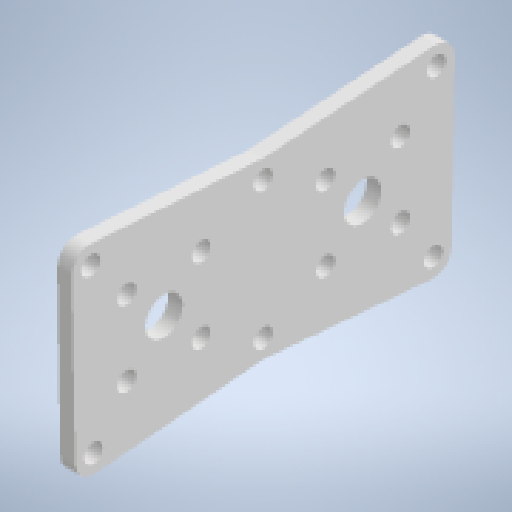
# Autodesk Inventor part: motorMountPlate2.0
Saved by Autodesk Inventor 2023 (Build 270158000, 158)
## iProperties
Created: 2022-09-08
Part Number: motorMountPlate2.0
Material: Generic
Document SubType Name: Modeling
Designer: deli
Density: 1 g/cm^3
Appearance: Default
Author: deli
Autodesk Inventor part; units mm, degrees
ref_plane "YZ Plane" through (0, 0, 0) normal (1, 0, 0) x (0, 1, 0)
ref_plane "XZ Plane" through (0, 0, 0) normal (0, 1, 0) x (-1, 0, 0)
ref_plane "XY Plane" through (0, 0, 0) normal (0, 0, 1) x (1, 0, 0)
sketch "Sketch1" plane through (0, 0, 0) normal (1, 0, 0) x (0, 1, 0)
  circle A0 centre (47.4062, -13.6361) radius 2 projected
  circle A1 centre (14.2614, -11.9601) radius 2 projected
  circle A2 centre (15.5288, -50.354) radius 2 projected
  circle A3 centre (44.494, -50.354) radius 2 projected
  circle A4 centre (47.4062, -87.072) radius 2 projected
  circle A5 centre (14.2614, -88.7479) radius 2 projected
  circle A6 centre (30.0114, -29.0628) radius 7 construction
  circle A7 centre (30.0114, -71.6453) radius 7 construction
  circle A8 centre (30.0114, -29.0628) radius 4
  circle A9 centre (30.0114, -71.6453) radius 4
  circle A10 centre (30.0114, -29.0628) radius 9.3137 construction
  circle A11 centre (30.0114, -71.6453) radius 9.3137 construction
  arc A12 (51.3935, -13.9551) -> (47.6082, -9.6412) centre (47.4062, -13.6361) ccw
  circle A13 centre (44.494, -50.354) radius 4 construction
  circle A14 centre (15.5288, -50.354) radius 4 construction
  arc A15 (14.4634, -7.9653) -> (10.2636, -12.0926) centre (14.2614, -11.9601) ccw
  arc A16 (10.2636, -88.6155) -> (14.4634, -92.7428) centre (14.2614, -88.7479) ccw
  arc A17 (47.6082, -91.0669) -> (51.3935, -86.7529) centre (47.4062, -87.072) ccw
  arc A18 (48.5067, -50.035) -> (48.5067, -50.6731) centre (52.494, -50.354) ccw
  arc A19 (11.5266, -50.4865) -> (11.5266, -50.2216) centre (7.5288, -50.354) ccw
  circle A20 centre (38.0114, -21.0628) radius 2
  circle A21 centre (38.0114, -37.0628) radius 2
  circle A22 centre (22.0114, -21.0628) radius 2
  circle A23 centre (22.0114, -37.0628) radius 2
  circle A24 centre (22.0114, -63.6453) radius 2
  circle A25 centre (22.0114, -79.6453) radius 2
  circle A26 centre (38.0114, -79.6453) radius 2
  circle A27 centre (38.0114, -63.6453) radius 2
  line L0 (38.0114, -21.0628) -> (38.0114, -37.0628) construction
  line L1 (38.0114, -37.0628) -> (22.0114, -37.0628) construction
  line L2 (22.0114, -37.0628) -> (22.0114, -21.0628) construction
  line L3 (22.0114, -21.0628) -> (38.0114, -21.0628) construction
  line L4 (38.0114, -63.6453) -> (38.0114, -79.6453) construction
  line L5 (38.0114, -79.6453) -> (22.0114, -79.6453) construction
  line L6 (22.0114, -79.6453) -> (22.0114, -63.6453) construction
  line L7 (38.0114, -63.6453) -> (22.0114, -63.6453) construction
  line L8 (51.3935, -13.9551) -> (48.5067, -50.035)
  line L9 (48.5067, -50.6731) -> (51.3935, -86.7529)
  line L10 (47.6082, -91.0669) -> (14.4634, -92.7428)
  line L11 (10.2636, -88.6155) -> (11.5266, -50.4865)
  line L12 (11.5266, -50.2216) -> (10.2636, -12.0926)
  line L13 (14.4634, -7.9653) -> (47.6082, -9.6412)
  point P0 (0, 0)
  dimension "d0" = 8
  dimension "d1" = 8
  dimension "d2" = 8
  dimension "d3" = 8
  dimension "d4" = 8
  dimension "d5" = 8
  dimension "d6" = 8
  dimension "d7" = 0
  dimension "d8" = 8
  dimension "d9" = 0
  dimension "d10" = 4
  dimension "d11" = 4
  dimension "d12" = 4
  dimension "d13" = 4
  dimension "d14" = 4
  dimension "d15" = 4
  dimension "d16" = 4
  dimension "d17" = 4
  dimension "d18" = 8
  dimension "d19" = 8
  dimension "d20" = 16
  dimension "d21" = 16
  dimension "d22" = 16
  dimension "d23" = 16
  constraints: 28 end point, 22 tangent, 20 centre point, 12 point on circle, 10 coincident, 3 perpendicular, 2 vertical, 1 collinear
  measures "d0" diameter of A12
  measures "d1" diameter of A18
  measures "d2" diameter of A15
  measures "d3" diameter of A14
  measures "d4" diameter of A19
  measures "d5" diameter of A16
  measures "d6" diameter of A17
  measures "d7" vertical distance of A18.centre A3.centre
  measures "d8" diameter of A13
  measures "d9" vertical distance of A14.centre A19.centre
  measures "d10" diameter of A22
  measures "d11" diameter of A23
  measures "d12" diameter of A21
  measures "d13" diameter of A20
  measures "d14" diameter of A27
  measures "d15" diameter of A24
  measures "d16" diameter of A25
  measures "d17" diameter of A26
  measures "d18" diameter of A8
  measures "d19" diameter of A9
  measures "d20" distance of L0.start L0.end
  measures "d21" distance of L2.end L0.start
  measures "d22" distance of L4.start L6.end
  measures "d23" distance of L4.start L4.end
extrude "Extrusion1" add sketch "Sketch1" along normal blind 3.175
equation "\"d1\" = d0"
equation "\"d2\" = d0"
equation "\"d3\" = d0"
equation "\"d4\" = d0"
equation "\"d5\" = d0"
equation "\"d6\" = d0"
equation "\"d8\" = d0"
equation "\"d11\" = d10"
equation "\"d12\" = d10"
equation "\"d13\" = d10"
equation "\"d14\" = d10"
equation "\"d15\" = d10"
equation "\"d16\" = d10"
equation "\"d17\" = d10"
equation "\"d18\" = d0"
equation "\"d19\" = d0"
equation "\"d21\" = d20"
equation "\"d22\" = d20"
equation "\"d23\" = d20"
body "Solid1"
